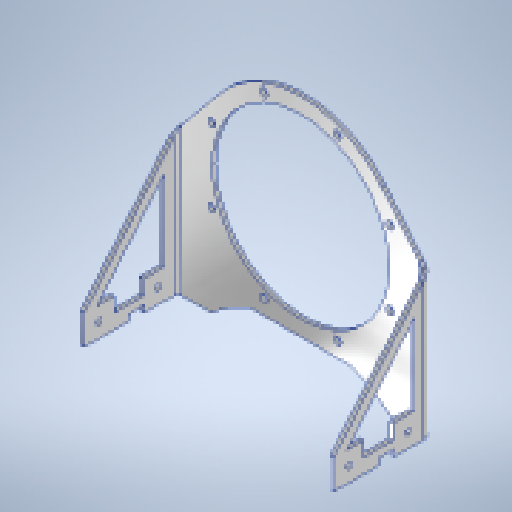
# Autodesk Inventor part: base_plate1
Saved by Autodesk Inventor 2024 (Build 280153000, 153)
## iProperties
Created: 2025-02-13
Part Number: base_plate1
Material: アルミニウム 6061
Document SubType Name: Sheet Metal
Designer: tanoue_kota
Density: 2.7 g/cm^3
Sheet Metal Rule: Default_mm
Appearance: アルミニウム - フラット
Flat Pattern Width: 18.3368 cm
Flat Pattern Length: 17.5225 cm
Flat Pattern Area: 321.307 cm^2
Sheet Metal Width: 183.368 mm
Sheet Metal Length: 175.225 mm
Sheet Metal Area: 32130.686 mm^2
Author: tanoue_kota
Autodesk Inventor part; units mm, degrees
ref_plane "YZ Plane" through (0, 0, 0) normal (1, 0, 0) x (0, 1, 0)
ref_plane "XZ Plane" through (0, 0, 0) normal (0, 1, 0) x (-1, 0, 0)
ref_plane "XY Plane" through (0, 0, 0) normal (0, 0, 1) x (1, 0, 0)
sketch "スケッチ5" plane through (0, 0, 0) normal (0, 0, 1) x (1, 0, 0)
  circle A0 centre (0, 0) radius 53
  circle A1 centre (0, 0) radius 40
  dimension "d28" = 106
  dimension "d29" = 80
  measures "d28" diameter of A0
  measures "d29" diameter of A1
extrude "プレート2" add sketch "スケッチ5" along normal blind 2
sketch "スケッチ6" plane through (0, 0, 2) normal (0, 0, 1) x (1, 0, 0)
  circle A0 centre (0, 0) radius 53
  line L0 (53, 0) -> (-53, 0)
  line L1 (-53, 0) -> (-53, -65)
  line L2 (-53, -65) -> (53, -65)
  line L3 (53, -65) -> (53, 0)
  line L4 (53, 0) -> (63, 0)
  line L5 (63, 0) -> (63, -65)
  line L6 (63, -65) -> (53, -65)
  line L7 (53, -65) -> (53, 0)
  line L8 (63, -65) -> (113, -65)
  line L9 (113, -65) -> (113, -50)
  line L10 (113, -50) -> (63, -50)
  line L11 (63, -50) -> (63, -65)
  line L12 (113, -50) -> (40.1612, 34.5843)
  line L13 (63, 0) -> (69.9431, 0)
  line L14 (0, 0) -> (0, -65)
  line L15 (-53, -65) -> (-53, 0)
  line L16 (-63, -65) -> (-53, -65)
  line L17 (-63, -65) -> (-113, -65)
  line L18 (-113, -65) -> (-113, -50)
  line L19 (-113, -50) -> (-40.1612, 34.5843)
  circle A1 centre (0, 0) radius 53
  point P0 (-40.1612, 34.5843)
  dimension "d80" = 65
  dimension "d81" = 10
  dimension "d82" = 50
  dimension "d83" = 15
  measures "d80" distance between parallel lines of L0 L2
  measures "d81" distance between parallel lines of L3 L5
  measures "d82" distance between parallel lines of L5 L9
  measures "d83" distance of L8.end L9.end
sheet face with bend "面3" sketch "スケッチ6" thickness 2 toward (0, 0, -1) bend radius 2
bend "曲げ2"
sketch "スケッチ9" plane through (0, 0, 2) normal (0, 0, 1) x (1, 0, 0)
  circle A0 centre (0, 0) radius 49
  line L0 (0, 0) -> (0, 53)
  arc A1 (40.1612, 34.5843) -> (-40.1612, 34.5843) centre (0, 0) ccw projected
  line L1 (0, 0) -> (18.7515, 45.2701)
  point P0 (53, 0)
  point P1 (53, 0)
  point P2 (-18.7515, 45.2701)
  point P3 (-45.2701, 18.7515)
  point P4 (-45.2701, -18.7515)
  point P5 (-18.7515, -45.2701)
  point P6 (18.7515, -45.2701)
  point P7 (45.2701, -18.7515)
  point P8 (45.2701, 18.7515)
  dimension "d51" = 98
  dimension "d52" = 22.5
  dimension "d55" = 360
  constraints: 4 end point, 2 coincident, 1 point on circle, 1 vertical, 12 other
  measures "d52" angle of L0 L1
hole "穴2" at (18.7515, 45.2701, 2) at (-18.7515, 45.2701, 2) at (-45.2701, 18.7515, 2) at (-45.2701, -18.7515, 2) at (-18.7515, -45.2701, 2) at (18.7515, -45.2701, 2) at (45.2701, -18.7515, 2) at (45.2701, 18.7515, 2) direction (0, 0, -1) diameter 4.1 end through all
sketch "スケッチ10" plane through (0, 0, 2) normal (0, 0, 1) x (1, 0, 0)
  arc A0 (40.1612, 34.5843) -> (-40.1612, 34.5843) centre (0, 0) ccw projected
  circle A1 centre (0, 0) radius 53
  line L0 (-40.1612, 34.5843) -> (-113, -50) projected
  line L1 (-63, 8.0627) -> (-63, -65)
  line L2 (-113, -65) -> (113, -65) projected
  line L3 (-113, -50) -> (-113, -65) projected
  dimension "d84" = 50
  constraints: 2 end point, 2 point on line, 1 coincident, 1 vertical, 3 other
  measures "d84" distance between parallel lines of L3 L1
fold "折り曲げ3" angle 90 bend radius 2 thickness 2 k factor 0.44 line from (-63, 8.0627, 2) to (-63, -65, 2) line at bend start moving side (-1, 0, 0) folds toward (0, 0, 1)
sketch "スケッチ11" plane through (0, 0, 2) normal (0, 0, 1) x (1, 0, 0)
  circle A0 centre (0, 0) radius 53
  line L0 (113, -50) -> (40.1612, 34.5843) projected
  line L1 (63, 8.0627) -> (63, -65)
  line L2 (-63, -65) -> (113, -65) projected
  line L3 (113, -65) -> (113, -50) projected
  dimension "d73" = 106
  dimension "d85" = 50
  constraints: 2 end point, 2 point on line, 1 coincident, 1 vertical, 2 other
  measures "d85" distance between parallel lines of L3 L1
fold "折り曲げ4" angle 90 bend radius 2 thickness 2 k factor 0.44 line from (63, 8.0627, 2) to (63, -65, 2) line at bend start moving side (1, 0, 0) folds toward (0, 0, 1)
sketch "スケッチ12" plane through (0, 0, 0) normal (0, 0, -1) x (-1, 0, 0)
  circle A0 centre (0, 0) radius 45
  dimension "d86" = 90
  constraints: 1 centre point, 1 coincident
  measures "d86" diameter of A0
extrude "押し出し3" cut sketch "スケッチ12" against normal blind 10
sketch "スケッチ13" plane through (67, -65, 49.4761) normal (1, 0, 0) x (0, 0, -1)
  line L0 (0, 0) -> (0, 15) projected
  line L1 (0, 7.5) -> (49.4761, 7.5)
  line L2 (49.4761, 0) -> (49.4761, 73.0627) projected
  point P0 (49.4761, 65)
  point P1 (7.5, 7.5)
  point P2 (37.5, 7.5)
  dimension "d89" = 7.5
  dimension "d90" = 30
  constraints: 3 point on line, 2 end point, 1 horizontal, 1 midpoint
  measures "d89" distance from line of L0 point (7.5, 7.5)
  measures "d90" distance of point (7.5, 7.5) point (37.5, 7.5)
hole "穴3" at (67, -57.5, 41.9761) at (67, -57.5, 11.9761) direction (-1, 0, 0) diameter 3.1 end through all
sketch "スケッチ14" plane through (0, 0, 2) normal (0, 0, 1) x (1, 0, 0)
  line L0 (0, 0) -> (0, -65)
  line L1 (-63, -65) -> (63, -65) projected
  arc A0 (0, -45.951) -> (-48, -65) centre (0, -115.951) ccw
  line L2 (-63, 8.0627) -> (-63, -65) projected
  arc A1 (48, -65) -> (0, -45.951) centre (0, -115.951) ccw
  line L3 (-63, -65) -> (63, -65)
  line L4 (-40.1612, 34.5843) -> (-63, 8.0627) projected
  line L5 (-58, 13.869) -> (-58, -65)
  line L6 (-58, -53) -> (0, -53)
  circle A2 centre (0, 0) radius 54
  line L7 (58, 13.869) -> (58, -65)
  line L8 (58, -53) -> (0, -53)
  line L9 (-25, -47.8644) -> (-25, -53)
  line L10 (25, -47.8644) -> (25, -53)
  point P0 (-47.7935, -53)
  point P1 (47.7935, -53)
  point P2 (10.3441, -53)
  point P3 (51, -17.7482)
  point P4 (-10.3441, -53)
  point P5 (-51, -17.7482)
  point P6 (25, -47.8644)
  point P7 (25, -53)
  point P8 (30.6133, -53)
  point P9 (-30.6133, -53)
  dimension "d102" = 108
  dimension "d98" = 15
  dimension "d99" = 70
  dimension "d100" = 5
  dimension "d101" = 12
  dimension "d105" = 25
  constraints: 16 end point, 11 point on line, 6 symmetric about line, 4 point on circle, 3 perpendicular, 2 centre point, 1 coincident, 1 horizontal, 1 midpoint, 4 other
  measures "d98" distance from line of L2 A0.end
  measures "d99" radius of A0
  measures "d100" distance between parallel lines of L2 L5
  measures "d101" distance between parallel lines of L1 L6
  measures "d105" distance between parallel lines of L0 L9
extrude "押し出し4" cut sketch "スケッチ14" against normal blind 10 contours L8 A2 L0 | L0 A2 L6 | A2 L8 A1 L1 L0 | L0 L1 A0 L6 A2
sketch "スケッチ15" plane through (-67, -65, 49.4761) normal (-1, 0, 0) x (0, 0, 1)
  line L0 (-45.4761, 67.8093) -> (0, 15) projected
  line L1 (0, 15) -> (-45.4761, 15)
  line L2 (-45.4761, 0) -> (-45.4761, 67.8093) projected
  circle A0 centre (-37.5, 7.5) radius 1.55 projected
  circle A1 centre (-7.5, 7.5) radius 1.55 projected
  line L3 (-37.5, 7.5) -> (-7.5, 7.5)
  line L4 (-30, 15) -> (-15, 15)
  line L5 (-15, 15) -> (-15, 7.5)
  line L6 (-15, 7.5) -> (-30, 7.5)
  line L7 (-30, 7.5) -> (-30, 15)
  line L8 (-40.4761, 62.003) -> (-40.4761, 15)
  line L9 (-40.4761, 54.3406) -> (-6.5984, 15)
  line L10 (-45.4761, 67.8093) -> (0, 15) projected
  point P0 (-49.4761, 65)
  point P1 (-30, 7.5)
  point P2 (-15, 15)
  dimension "d106" = 7.5
  dimension "d107" = 7.5
  dimension "d108" = 5
  dimension "d109" = 5
  constraints: 16 end point, 7 point on line, 3 horizontal, 3 parallel, 2 perpendicular
  measures "d106" distance from line of L3.start L7
  measures "d107" distance from line of L3.end L5
  measures "d108" distance between parallel lines of L2 L8
  measures "d109" distance between parallel lines of L0 L9
extrude "押し出し5" cut sketch "スケッチ15" against normal blind 150 contours L9 L1 L8 | L1 L5 L3 L7
sketch "スケッチ16" plane through (-67, -65, 49.4761) normal (-1, 0, 0) x (0, 0, 1)
  line L0 (-45.4761, 0) -> (0, 0) projected
  line L1 (-31.2, 0) -> (-22.7, 0)
  line L2 (-22.7, 0) -> (-22.7, 4.3)
  line L3 (-22.7, 4.3) -> (-31.2, 4.3)
  line L4 (-31.2, 4.3) -> (-31.2, 0)
  line L5 (0, 15) -> (0, 0) projected
  point P0 (-49.4761, 65)
  point P1 (-22.7, 0)
  dimension "d112" = 8.5
  dimension "d113" = 4.3
  dimension "d114" = 22.7
  constraints: 8 end point, 2 parallel, 1 horizontal, 1 perpendicular, 1 point on line
  measures "d112" distance of L2.end L3.end
  measures "d113" distance of L1.end L2.end
  measures "d114" distance between parallel lines of L5 L2
extrude "押し出し6" cut sketch "スケッチ16" against normal blind 150
sketch "スケッチ1" plane through (-20.4327, -48.0365, 0) normal (0, 0, 1) x (0.9998505, 0.0172924, 0)
  line L0 (19.7844, 45.962) -> (73.1579, 0) projected
  line L1 (158.3292, 98.9056) -> (104.9557, 144.8676) projected
  line L2 (93.6917, 131.7872) -> (115.7474, 157.3994) projected
  line L3 (8.9927, 33.4301) -> (31.0484, 59.0423) projected
  point P0 (22.0576, 44.0043)
  point P1 (107.229, 142.91)
  point P2 (25.8464, 40.7417)
  point P3 (111.0178, 139.6473)
  point P4 (29.6352, 37.479)
  point P5 (114.8066, 136.3846)
  point P6 (33.424, 34.2163)
  point P7 (118.5954, 133.1219)
  point P8 (37.2128, 30.9536)
  point P9 (122.3842, 129.8593)
  point P10 (41.0016, 27.691)
  point P11 (126.173, 126.5966)
  point P12 (44.7904, 24.4283)
  point P13 (129.9618, 123.3339)
  point P14 (48.5792, 21.1656)
  point P15 (133.7506, 120.0713)
  point P16 (52.368, 17.903)
  point P17 (137.5394, 116.8086)
  point P18 (56.1568, 14.6403)
  point P19 (141.3282, 113.5459)
  point P20 (59.9456, 11.3776)
  point P21 (145.117, 110.2832)
  point P22 (63.7344, 8.1149)
  point P23 (148.9057, 107.0206)
  point P24 (67.5232, 4.8523)
  point P25 (152.6945, 103.7579)
  point P26 (71.312, 1.5896)
  point P27 (156.4833, 100.4952)
  dimension "d0" = 3
  dimension "d1" = 3
  dimension "d4" = 5
  constraints: 2 point on line, 27 other
  measures "d0" distance from line of L2 point (107.229, 142.91)
  measures "d1" distance from line of L3 point (22.058, 44.004)
  measures "d4" distance of point (22.058, 44.004) point (25.846, 40.742)
equation "\"d30\" = Thickness"
equation "\"d67\" = BendReliefWidth"
equation "\"d68\" = BendReliefDepth"
equation "\"d69\" = MinimumRemnant"
equation "\"d70\" = TransitionRadius"
equation "\"d72\" = BendRadius"
equation "\"d74\" = BendReliefWidth"
equation "\"d75\" = BendReliefDepth"
equation "\"d76\" = MinimumRemnant"
equation "\"d77\" = TransitionRadius"
equation "\"d79\" = BendRadius"
equation "\"d96\" = Thickness"
equation "\"d34\" = BendRadius"
equation "\"d35\" = BendReliefWidth"
equation "\"d37\" = MinimumRemnant"
equation "\"d36\" = BendReliefDepth"
equation "\"d38\" = TransitionRadius"
equation "\"BendRadius\" = Thickness"
equation "\"BendReliefWidth\" = Thickness"
equation "\"BendReliefDepth\" = 0.5 * Thickness"
equation "\"CornerReliefSize\" = 4 * Thickness"
equation "\"MinimumRemnant\" = 2 * Thickness"
equation "\"TransitionRadius\" = BendRadius"
equation "\"JacobiRadiusSize\" = BendRadius"
equation "\"GapSize\" = Thickness"
equation "\"Thickness\" = 2"
